Autodesk Fusion 360 part; units mm, degrees
note: some values were not read from the file. Chosen so that the rebuilt part matches the saved one: a direction. Set by a fixed rule: which sketch regions a step uses.
(part 5 of 6)
  spline S19 degree 5 poles (-3.1053, -47.8876) (-3.107, -47.8816) (-3.1103, -47.8695) (-3.1154, -47.8514) (-3.1223, -47.8272) (-3.1309, -47.7972) (-3.1397, -47.7672) (-3.1486, -47.7373) (-3.1576, -47.7075) (-3.1668, -47.6777) (-3.176, -47.6481) (-3.1854, -47.6185) (-3.1949, -47.589) (-3.2046, -47.5596) (-3.2143, -47.5303) (-3.2242, -47.5011) (-3.2342, -47.472) (-3.2443, -47.4429) (-3.2546, -47.414) (-3.2649, -47.3851) (-3.2754, -47.3563) (-3.2861, -47.3277) (-3.2968, -47.2991) (-3.3077, -47.2706) (-3.3187, -47.2422) (-3.3298, -47.2139) (-3.3411, -47.1858) (-3.3525, -47.1577) (-3.364, -47.1297) (-3.3756, -47.1018) (-3.3874, -47.074) (-3.3993, -47.0463) (-3.4114, -47.0188) (-3.4236, -46.9913) (-3.4359, -46.964) (-3.4483, -46.9367) (-3.4609, -46.9096) (-3.4736, -46.8826) (-3.4865, -46.8557) (-3.4995, -46.8289) (-3.5126, -46.8023) (-3.5259, -46.7758) (-3.5394, -46.7494) (-3.5529, -46.7231) (-3.5667, -46.6969) (-3.5805, -46.6709) (-3.5946, -46.645) (-3.6087, -46.6193) (-3.623, -46.5936) (-3.6375, -46.5682) (-3.6522, -46.5428) (-3.667, -46.5177) (-3.6819, -46.4926) (-3.6971, -46.4678) (-3.7124, -46.4431) (-3.7279, -46.4186) (-3.7436, -46.3942) (-3.7594, -46.3699) (-3.7753, -46.3458) (-3.7915, -46.3219) (-3.8078, -46.2982) (-3.8245, -46.2748) (-3.8414, -46.2516) (-3.8585, -46.2287) (-3.8759, -46.2061) (-3.8935, -46.1836) (-3.9112, -46.1612) (-3.9291, -46.139) (-3.9471, -46.117) (-3.9654, -46.0954) (-3.9844, -46.0743) (-4.0001, -46.0581) (-4.0123, -46.0463) (-4.0207, -46.0387) (-4.0249, -46.0349) knots -1 -1 -1 -1 -1 -1 -0.98571429 -0.97142857 -0.95714286 -0.94285714 -0.92857143 -0.91428571 -0.9 -0.88571429 -0.87142857 -0.85714286 -0.84285714 -0.82857143 -0.81428571 -0.8 -0.78571429 -0.77142857 -0.75714286 -0.74285714 -0.72857143 -0.71428571 -0.7 -0.68571429 -0.67142857 -0.65714286 -0.64285714 -0.62857143 -0.61428571 -0.6 -0.58571429 -0.57142857 -0.55714286 -0.54285714 -0.52857143 -0.51428571 -0.5 -0.48571429 -0.47142857 -0.45714286 -0.44285714 -0.42857143 -0.41428571 -0.4 -0.38571429 -0.37142857 -0.35714286 -0.34285714 -0.32857143 -0.31428571 -0.3 -0.28571429 -0.27142857 -0.25714286 -0.24285714 -0.22857143 -0.21428571 -0.2 -0.18571429 -0.17142857 -0.15714286 -0.14285714 -0.12857143 -0.11428571 -0.1 -0.08571429 -0.07142857 -0.05714286 -0.04285714 -0.02857143 -0.01428571 0 0 0 0 0 0
  line L19 (-4.0249, -46.0349) -> (-4.3883, -45.7105)
  arc A39 (-4.397, -45.57) -> (-4.3883, -45.7105) centre (-4.3217, -45.6359) ccw
  arc A40 (-4.397, -45.57) -> (-3.7561, -44.7724) centre (-13.5, -37.5997) ccw
  arc A41 (-3.6171, -44.7506) -> (-3.7561, -44.7724) centre (-3.6756, -44.8317) ccw
  line L20 (-3.6171, -44.7506) -> (-3.222, -45.0357)
  spline S20 degree 5 poles (-3.222, -45.0357) (-3.2174, -45.039) (-3.2081, -45.0455) (-3.194, -45.0549) (-3.1748, -45.0668) (-3.1502, -45.0807) (-3.1251, -45.094) (-3.0997, -45.1068) (-3.0742, -45.1194) (-3.0485, -45.1319) (-3.0228, -45.1442) (-2.9969, -45.1563) (-2.9708, -45.1682) (-2.9446, -45.1797) (-2.9181, -45.1909) (-2.8915, -45.2018) (-2.8646, -45.2124) (-2.8377, -45.2228) (-2.8106, -45.233) (-2.7834, -45.243) (-2.7561, -45.2529) (-2.7287, -45.2625) (-2.7012, -45.272) (-2.6735, -45.2812) (-2.6457, -45.2902) (-2.6178, -45.2991) (-2.5898, -45.3077) (-2.5617, -45.3162) (-2.5335, -45.3245) (-2.5052, -45.3326) (-2.4768, -45.3405) (-2.4483, -45.3483) (-2.4198, -45.3559) (-2.3911, -45.3633) (-2.3623, -45.3706) (-2.3335, -45.3777) (-2.3045, -45.3846) (-2.2755, -45.3914) (-2.2464, -45.398) (-2.2172, -45.4044) (-2.1879, -45.4107) (-2.1585, -45.4169) (-2.1291, -45.4229) (-2.0996, -45.4287) (-2.07, -45.4344) (-2.0403, -45.4399) (-2.0106, -45.4452) (-1.9808, -45.4505) (-1.9509, -45.4555) (-1.921, -45.4605) (-1.8909, -45.4652) (-1.8608, -45.4699) (-1.8307, -45.4744) (-1.8005, -45.4787) (-1.7702, -45.4829) (-1.7398, -45.487) (-1.7094, -45.4909) (-1.6789, -45.4946) (-1.6484, -45.4983) (-1.6178, -45.5018) (-1.5871, -45.5051) (-1.5564, -45.5083) (-1.5256, -45.5114) (-1.4948, -45.5143) (-1.4639, -45.5171) (-1.4329, -45.5198) (-1.4019, -45.5223) (-1.3709, -45.5247) (-1.3397, -45.527) (-1.3086, -45.5291) (-1.2773, -45.5311) (-1.2523, -45.5326) (-1.2335, -45.5336) (-1.221, -45.5343) (-1.2147, -45.5346) knots 0 0 0 0 0 0 0.01428571 0.02857143 0.04285714 0.05714286 0.07142857 0.08571429 0.1 0.11428571 0.12857143 0.14285714 0.15714286 0.17142857 0.18571429 0.2 0.21428571 0.22857143 0.24285714 0.25714286 0.27142857 0.28571429 0.3 0.31428571 0.32857143 0.34285714 0.35714286 0.37142857 0.38571429 0.4 0.41428571 0.42857143 0.44285714 0.45714286 0.47142857 0.48571429 0.5 0.51428571 0.52857143 0.54285714 0.55714286 0.57142857 0.58571429 0.6 0.61428571 0.62857143 0.64285714 0.65714286 0.67142857 0.68571429 0.7 0.71428571 0.72857143 0.74285714 0.75714286 0.77142857 0.78571429 0.8 0.81428571 0.82857143 0.84285714 0.85714286 0.87142857 0.88571429 0.9 0.91428571 0.92857143 0.94285714 0.95714286 0.97142857 0.98571429 1 1 1 1 1 1
  arc A42 (-1.2147, -45.5346) -> (-0.7968, -44.8467) centre (-13.5, -37.5997) ccw
  spline S21 degree 5 poles (-0.7968, -44.8467) (-0.8, -44.8413) (-0.8064, -44.8305) (-0.8159, -44.8143) (-0.8288, -44.7928) (-0.8449, -44.766) (-0.8612, -44.7393) (-0.8775, -44.7127) (-0.894, -44.6863) (-0.9105, -44.6599) (-0.9271, -44.6337) (-0.9438, -44.6075) (-0.9606, -44.5815) (-0.9776, -44.5556) (-0.9946, -44.5298) (-1.0117, -44.5041) (-1.0289, -44.4786) (-1.0462, -44.4532) (-1.0636, -44.4278) (-1.081, -44.4027) (-1.0986, -44.3776) (-1.1163, -44.3526) (-1.1341, -44.3278) (-1.152, -44.3031) (-1.1699, -44.2785) (-1.188, -44.2541) (-1.2062, -44.2298) (-1.2245, -44.2056) (-1.2428, -44.1816) (-1.2613, -44.1576) (-1.2799, -44.1339) (-1.2985, -44.1102) (-1.3173, -44.0867) (-1.3362, -44.0633) (-1.3552, -44.0401) (-1.3742, -44.017) (-1.3934, -43.9941) (-1.4127, -43.9713) (-1.4321, -43.9486) (-1.4516, -43.9261) (-1.4712, -43.9038) (-1.4909, -43.8816) (-1.5107, -43.8596) (-1.5306, -43.8377) (-1.5506, -43.816) (-1.5707, -43.7945) (-1.591, -43.7731) (-1.6113, -43.7519) (-1.6318, -43.7308) (-1.6524, -43.71) (-1.6731, -43.6893) (-1.6939, -43.6688) (-1.7148, -43.6485) (-1.7359, -43.6284) (-1.7571, -43.6086) (-1.7784, -43.5889) (-1.7998, -43.5694) (-1.8214, -43.55) (-1.843, -43.5309) (-1.8648, -43.512) (-1.8867, -43.4933) (-1.9089, -43.475) (-1.9312, -43.457) (-1.9537, -43.4393) (-1.9764, -43.4219) (-1.9992, -43.4048) (-2.0221, -43.3878) (-2.045, -43.3709) (-2.0681, -43.3543) (-2.0915, -43.3382) (-2.1152, -43.3227) (-2.1346, -43.3111) (-2.1495, -43.3029) (-2.1595, -43.2977) (-2.1645, -43.2952) knots -1 -1 -1 -1 -1 -1 -0.98571429 -0.97142857 -0.95714286 -0.94285714 -0.92857143 -0.91428571 -0.9 -0.88571429 -0.87142857 -0.85714286 -0.84285714 -0.82857143 -0.81428571 -0.8 -0.78571429 -0.77142857 -0.75714286 -0.74285714 -0.72857143 -0.71428571 -0.7 -0.68571429 -0.67142857 -0.65714286 -0.64285714 -0.62857143 -0.61428571 -0.6 -0.58571429 -0.57142857 -0.55714286 -0.54285714 -0.52857143 -0.51428571 -0.5 -0.48571429 -0.47142857 -0.45714286 -0.44285714 -0.42857143 -0.41428571 -0.4 -0.38571429 -0.37142857 -0.35714286 -0.34285714 -0.32857143 -0.31428571 -0.3 -0.28571429 -0.27142857 -0.25714286 -0.24285714 -0.22857143 -0.21428571 -0.2 -0.18571429 -0.17142857 -0.15714286 -0.14285714 -0.12857143 -0.11428571 -0.1 -0.08571429 -0.07142857 -0.05714286 -0.04285714 -0.02857143 -0.01428571 0 0 0 0 0 0
  line L21 (-2.1645, -43.2952) -> (-2.5996, -43.0759)
  arc A43 (-2.6443, -42.9424) -> (-2.5996, -43.0759) centre (-2.5546, -42.9866) ccw
  arc A44 (-2.6443, -42.9424) -> (-2.2317, -42.0061) centre (-13.5, -37.5997) ccw
  arc A45 (-2.1031, -41.9491) -> (-2.2317, -42.0061) centre (-2.1386, -42.0425) ccw
  line L22 (-2.1031, -41.9491) -> (-1.6476, -42.1221)
  spline S22 degree 5 poles (-1.6476, -42.1221) (-1.6423, -42.1241) (-1.6317, -42.128) (-1.6157, -42.1335) (-1.594, -42.14) (-1.5666, -42.147) (-1.5389, -42.1534) (-1.5111, -42.1592) (-1.4832, -42.1648) (-1.4552, -42.1702) (-1.4271, -42.1755) (-1.399, -42.1805) (-1.3707, -42.1851) (-1.3424, -42.1895) (-1.3139, -42.1934) (-1.2854, -42.1971) (-1.2567, -42.2004) (-1.228, -42.2034) (-1.1992, -42.2063) (-1.1703, -42.2089) (-1.1414, -42.2114) (-1.1124, -42.2136) (-1.0834, -42.2156) (-1.0543, -42.2174) (-1.0251, -42.2189) (-0.9959, -42.2202) (-0.9666, -42.2213) (-0.9373, -42.2222) (-0.9079, -42.2229) (-0.8785, -42.2234) (-0.849, -42.2238) (-0.8194, -42.2239) (-0.7899, -42.2238) (-0.7602, -42.2236) (-0.7306, -42.2232) (-0.7009, -42.2225) (-0.6711, -42.2218) (-0.6413, -42.2208) (-0.6115, -42.2196) (-0.5816, -42.2183) (-0.5517, -42.2168) (-0.5218, -42.2151) (-0.4918, -42.2133) (-0.4618, -42.2113) (-0.4317, -42.2091) (-0.4016, -42.2067) (-0.3715, -42.2042) (-0.3414, -42.2016) (-0.3112, -42.1987) (-0.281, -42.1957) (-0.2508, -42.1926) (-0.2205, -42.1893) (-0.1902, -42.1858) (-0.1599, -42.1822) (-0.1295, -42.1784) (-0.0992, -42.1744) (-0.0688, -42.1704) (-0.0384, -42.1661) (-0.0079, -42.1617) (0.0225, -42.1572) (0.053, -42.1525) (0.0835, -42.1476) (0.1141, -42.1426) (0.1446, -42.1375) (0.1752, -42.1322) (0.2058, -42.1267) (0.2364, -42.1212) (0.267, -42.1154) (0.2976, -42.1095) (0.3283, -42.1035) (0.359, -42.0974) (0.3835, -42.0923) (0.4019, -42.0885) (0.4142, -42.0859) (0.4204, -42.0846) knots 0 0 0 0 0 0 0.01428571 0.02857143 0.04285714 0.05714286 0.07142857 0.08571429 0.1 0.11428571 0.12857143 0.14285714 0.15714286 0.17142857 0.18571429 0.2 0.21428571 0.22857143 0.24285714 0.25714286 0.27142857 0.28571429 0.3 0.31428571 0.32857143 0.34285714 0.35714286 0.37142857 0.38571429 0.4 0.41428571 0.42857143 0.44285714 0.45714286 0.47142857 0.48571429 0.5 0.51428571 0.52857143 0.54285714 0.55714286 0.57142857 0.58571429 0.6 0.61428571 0.62857143 0.64285714 0.65714286 0.67142857 0.68571429 0.7 0.71428571 0.72857143 0.74285714 0.75714286 0.77142857 0.78571429 0.8 0.81428571 0.82857143 0.84285714 0.85714286 0.87142857 0.88571429 0.9 0.91428571 0.92857143 0.94285714 0.95714286 0.97142857 0.98571429 1 1 1 1 1 1
  arc A46 (0.4204, -42.0846) -> (0.646, -41.312) centre (-13.5, -37.5997) ccw
  spline S23 degree 5 poles (0.646, -41.312) (0.6415, -41.3076) (0.6326, -41.2988) (0.6191, -41.2856) (0.6012, -41.2681) (0.5786, -41.2464) (0.556, -41.2249) (0.5334, -41.2034) (0.5106, -41.1821) (0.4878, -41.1609) (0.465, -41.1399) (0.4421, -41.119) (0.4191, -41.0982) (0.3961, -41.0775) (0.373, -41.057) (0.3498, -41.0367) (0.3266, -41.0164) (0.3033, -40.9963) (0.2799, -40.9764) (0.2565, -40.9566) (0.233, -40.9369) (0.2095, -40.9174) (0.1859, -40.898) (0.1622, -40.8788) (0.1385, -40.8597) (0.1147, -40.8408) (0.0909, -40.822) (0.067, -40.8034) (0.043, -40.7849) (0.019, -40.7666) (-0.0051, -40.7484) (-0.0293, -40.7304) (-0.0535, -40.7126) (-0.0777, -40.6949) (-0.1021, -40.6773) (-0.1265, -40.66) (-0.1509, -40.6428) (-0.1755, -40.6258) (-0.2001, -40.6089) (-0.2247, -40.5922) (-0.2494, -40.5757) (-0.2742, -40.5594) (-0.299, -40.5432) (-0.3239, -40.5273) (-0.3489, -40.5115) (-0.3739, -40.4959) (-0.399, -40.4805) (-0.4241, -40.4652) (-0.4493, -40.4502) (-0.4746, -40.4354) (-0.5, -40.4208) (-0.5254, -40.4064) (-0.5508, -40.3922) (-0.5764, -40.3782) (-0.602, -40.3645) (-0.6277, -40.351) (-0.6534, -40.3377) (-0.6793, -40.3246) (-0.7051, -40.3117) (-0.7311, -40.2991) (-0.7571, -40.2868) (-0.7832, -40.2748) (-0.8094, -40.2632) (-0.8357, -40.2519) (-0.8621, -40.241) (-0.8886, -40.2303) (-0.9151, -40.2198) (-0.9417, -40.2095) (-0.9683, -40.1995) (-0.995, -40.1899) (-1.0219, -40.1811) (-1.0437, -40.1749) (-1.0601, -40.1709) (-1.0712, -40.1684) (-1.0767, -40.1673) knots -1 -1 -1 -1 -1 -1 -0.98571429 -0.97142857 -0.95714286 -0.94285714 -0.92857143 -0.91428571 -0.9 -0.88571429 -0.87142857 -0.85714286 -0.84285714 -0.82857143 -0.81428571 -0.8 -0.78571429 -0.77142857 -0.75714286 -0.74285714 -0.72857143 -0.71428571 -0.7 -0.68571429 -0.67142857 -0.65714286 -0.64285714 -0.62857143 -0.61428571 -0.6 -0.58571429 -0.57142857 -0.55714286 -0.54285714 -0.52857143 -0.51428571 -0.5 -0.48571429 -0.47142857 -0.45714286 -0.44285714 -0.42857143 -0.41428571 -0.4 -0.38571429 -0.37142857 -0.35714286 -0.34285714 -0.32857143 -0.31428571 -0.3 -0.28571429 -0.27142857 -0.25714286 -0.24285714 -0.22857143 -0.21428571 -0.2 -0.18571429 -0.17142857 -0.15714286 -0.14285714 -0.12857143 -0.11428571 -0.1 -0.08571429 -0.07142857 -0.05714286 -0.04285714 -0.02857143 -0.01428571 0 0 0 0 0 0
  line L23 (-1.0767, -40.1673) -> (-1.5537, -40.068)
  arc A47 (-1.6314, -39.9507) -> (-1.5537, -40.068) centre (-1.5333, -39.9701) ccw
  arc A48 (-1.6314, -39.9507) -> (-1.4752, -38.9395) centre (-13.5, -37.5997) ccw
  arc A49 (-1.3657, -38.8511) -> (-1.4752, -38.9395) centre (-1.3758, -38.9506) ccw
  line L24 (-1.3657, -38.8511) -> (-0.881, -38.9004)
  spline S24 degree 5 poles (-0.881, -38.9004) (-0.8754, -38.901) (-0.8641, -38.902) (-0.8472, -38.9031) (-0.8246, -38.9038) (-0.7963, -38.9035) (-0.7679, -38.9025) (-0.7395, -38.9009) (-0.7111, -38.8991) (-0.6827, -38.8971) (-0.6542, -38.8949) (-0.6257, -38.8924) (-0.5972, -38.8896) (-0.5687, -38.8865) (-0.5402, -38.8829) (-0.5117, -38.879) (-0.4832, -38.8748) (-0.4546, -38.8703) (-0.4261, -38.8656) (-0.3975, -38.8607) (-0.3689, -38.8556) (-0.3404, -38.8502) (-0.3118, -38.8447) (-0.2832, -38.8388) (-0.2547, -38.8328) (-0.2261, -38.8265) (-0.1975, -38.82) (-0.1689, -38.8132) (-0.1404, -38.8063) (-0.1118, -38.7992) (-0.0832, -38.7919) (-0.0547, -38.7844) (-0.0261, -38.7767) (0.0024, -38.7688) (0.031, -38.7607) (0.0595, -38.7524) (0.088, -38.7439) (0.1166, -38.7352) (0.1451, -38.7264) (0.1736, -38.7174) (0.2021, -38.7082) (0.2306, -38.6988) (0.2591, -38.6893) (0.2875, -38.6796) (0.316, -38.6697) (0.3444, -38.6597) (0.3729, -38.6494) (0.4013, -38.6391) (0.4297, -38.6285) (0.4581, -38.6178) (0.4865, -38.6069) (0.5149, -38.5959) (0.5432, -38.5847) (0.5716, -38.5734) (0.5999, -38.5618) (0.6282, -38.5502) (0.6565, -38.5384) (0.6848, -38.5264) (0.7131, -38.5143) (0.7413, -38.502) (0.7696, -38.4896) (0.7978, -38.477) (0.826, -38.4642) (0.8541, -38.4514) (0.8823, -38.4383) (0.9104, -38.4252) (0.9386, -38.4119) (0.9666, -38.3984) (0.9947, -38.3848) (1.0228, -38.371) (1.0508, -38.3571) (1.0732, -38.3459) (1.09, -38.3374) (1.1012, -38.3317) (1.1068, -38.3289) knots 0 0 0 0 0 0 0.01428571 0.02857143 0.04285714 0.05714286 0.07142857 0.08571429 0.1 0.11428571 0.12857143 0.14285714 0.15714286 0.17142857 0.18571429 0.2 0.21428571 0.22857143 0.24285714 0.25714286 0.27142857 0.28571429 0.3 0.31428571 0.32857143 0.34285714 0.35714286 0.37142857 0.38571429 0.4 0.41428571 0.42857143 0.44285714 0.45714286 0.47142857 0.48571429 0.5 0.51428571 0.52857143 0.54285714 0.55714286 0.57142857 0.58571429 0.6 0.61428571 0.62857143 0.64285714 0.65714286 0.67142857 0.68571429 0.7 0.71428571 0.72857143 0.74285714 0.75714286 0.77142857 0.78571429 0.8 0.81428571 0.82857143 0.84285714 0.85714286 0.87142857 0.88571429 0.9 0.91428571 0.92857143 0.94285714 0.95714286 0.97142857 0.98571429 1 1 1 1 1 1
  arc A50 (1.1068, -38.3289) -> (1.1248, -37.5242) centre (-13.5, -37.5997) ccw
  spline S25 degree 5 poles (1.1248, -37.5242) (1.1193, -37.5211) (1.1084, -37.5149) (1.092, -37.5057) (1.0701, -37.4935) (1.0427, -37.4784) (1.0153, -37.4634) (0.9879, -37.4485) (0.9604, -37.4338) (0.9329, -37.4193) (0.9054, -37.4048) (0.8779, -37.3906) (0.8503, -37.3764) (0.8227, -37.3625) (0.7951, -37.3486) (0.7674, -37.335) (0.7398, -37.3214) (0.7121, -37.3081) (0.6843, -37.2948) (0.6566, -37.2818) (0.6288, -37.2688) (0.601, -37.2561) (0.5732, -37.2435) (0.5454, -37.231) (0.5176, -37.2187) (0.4897, -37.2066) (0.4618, -37.1946) (0.4339, -37.1828) (0.4059, -37.1712) (0.378, -37.1597) (0.35, -37.1484) (0.322, -37.1372) (0.294, -37.1263) (0.266, -37.1155) (0.2379, -37.1048) (0.2099, -37.0944) (0.1818, -37.0841) (0.1537, -37.074) (0.1256, -37.0641) (0.0975, -37.0543) (0.0693, -37.0448) (0.0412, -37.0354) (0.013, -37.0263) (-0.0152, -37.0173) (-0.0434, -37.0085) (-0.0716, -36.9999) (-0.0998, -36.9915) (-0.128, -36.9833) (-0.1563, -36.9753) (-0.1845, -36.9675) (-0.2128, -36.96) (-0.2411, -36.9526) (-0.2693, -36.9455) (-0.2976, -36.9387) (-0.3259, -36.9321) (-0.3542, -36.9257) (-0.3825, -36.9195) (-0.4109, -36.9135) (-0.4392, -36.9078) (-0.4675, -36.9023) (-0.4958, -36.8971) (-0.5241, -36.8923) (-0.5525, -36.8879) (-0.5808, -36.8838) (-0.6092, -36.8801) (-0.6375, -36.8766) (-0.6658, -36.8733) (-0.6941, -36.8702) (-0.7224, -36.8674) (-0.7507, -36.8651) (-0.779, -36.8636) (-0.8016, -36.8632) (-0.8185, -36.8636) (-0.8298, -36.8641) (-0.8355, -36.8644) knots -1 -1 -1 -1 -1 -1 -0.98571429 -0.97142857 -0.95714286 -0.94285714 -0.92857143 -0.91428571 -0.9 -0.88571429 -0.87142857 -0.85714286 -0.84285714 -0.82857143 -0.81428571 -0.8 -0.78571429 -0.77142857 -0.75714286 -0.74285714 -0.72857143 -0.71428571 -0.7 -0.68571429 -0.67142857 -0.65714286 -0.64285714 -0.62857143 -0.61428571 -0.6 -0.58571429 -0.57142857 -0.55714286 -0.54285714 -0.52857143 -0.51428571 -0.5 -0.48571429 -0.47142857 -0.45714286 -0.44285714 -0.42857143 -0.41428571 -0.4 -0.38571429 -0.37142857 -0.35714286 -0.34285714 -0.32857143 -0.31428571 -0.3 -0.28571429 -0.27142857 -0.25714286 -0.24285714 -0.22857143 -0.21428571 -0.2 -0.18571429 -0.17142857 -0.15714286 -0.14285714 -0.12857143 -0.11428571 -0.1 -0.08571429 -0.07142857 -0.05714286 -0.04285714 -0.02857143 -0.01428571 0 0 0 0 0 0
  line L25 (-0.8355, -36.8644) -> (-1.3219, -36.892)
  arc A51 (-1.4273, -36.7988) -> (-1.3219, -36.892) centre (-1.3276, -36.7921) ccw
  arc A52 (-1.4273, -36.7988) -> (-1.5382, -35.7816) centre (-13.5, -37.5997) ccw
  arc A53 (-1.4553, -35.6679) -> (-1.5382, -35.7816) centre (-1.4393, -35.7666) ccw
  line L26 (-1.4553, -35.6679) -> (-0.9743, -35.5901)
  spline S26 degree 5 poles (-0.9743, -35.5901) (-0.9688, -35.5892) (-0.9576, -35.5872) (-0.941, -35.5839) (-0.919, -35.5787) (-0.8917, -35.5711) (-0.8646, -35.5628) (-0.8376, -35.5539) (-0.8106, -35.5448) (-0.7836, -35.5355) (-0.7567, -35.526) (-0.7298, -35.5162) (-0.703, -35.5062) (-0.6763, -35.4958) (-0.6497, -35.485) (-0.6232, -35.4738) (-0.5967, -35.4624) (-0.5703, -35.4506) (-0.5439, -35.4387) (-0.5176, -35.4266) (-0.4913, -35.4142) (-0.4651, -35.4017) (-0.439, -35.3889) (-0.4129, -35.3759) (-0.3868, -35.3626) (-0.3609, -35.3491) (-0.335, -35.3355) (-0.3091, -35.3216) (-0.2833, -35.3075) (-0.2576, -35.2932) (-0.2319, -35.2787) (-0.2062, -35.2641) (-0.1806, -35.2493) (-0.1551, -35.2342) (-0.1296, -35.219) (-0.1042, -35.2036) (-0.0788, -35.1881) (-0.0535, -35.1723) (-0.0283, -35.1564) (-0.0031, -35.1403) (0.0221, -35.1241) (0.0472, -35.1077) (0.0722, -35.0911) (0.0972, -35.0743) (0.1222, -35.0574) (0.147, -35.0403) (0.1719, -35.0231) (0.1966, -35.0057) (0.2214, -34.9882) (0.246, -34.9705) (0.2706, -34.9526) (0.2952, -34.9346) (0.3197, -34.9165) (0.3441, -34.8982) (0.3685, -34.8797) (0.3928, -34.8611) (0.4171, -34.8424) (0.4413, -34.8235) (0.4655, -34.8045) (0.4896, -34.7853) (0.5136, -34.766) (0.5376, -34.7465) (0.5616, -34.727) (0.5855, -34.7072) (0.6093, -34.6874) (0.6331, -34.6673) (0.6568, -34.6472) (0.6804, -34.6269) (0.704, -34.6065) (0.7276, -34.586) (0.751, -34.5653) (0.7698, -34.5487) (0.7838, -34.5361) (0.7932, -34.5277) (0.7978, -34.5235) knots 0 0 0 0 0 0 0.01428571 0.02857143 0.04285714 0.05714286 0.07142857 0.08571429 0.1 0.11428571 0.12857143 0.14285714 0.15714286 0.17142857 0.18571429 0.2 0.21428571 0.22857143 0.24285714 0.25714286 0.27142857 0.28571429 0.3 0.31428571 0.32857143 0.34285714 0.35714286 0.37142857 0.38571429 0.4 0.41428571 0.42857143 0.44285714 0.45714286 0.47142857 0.48571429 0.5 0.51428571 0.52857143 0.54285714 0.55714286 0.57142857 0.58571429 0.6 0.61428571 0.62857143 0.64285714 0.65714286 0.67142857 0.68571429 0.7 0.71428571 0.72857143 0.74285714 0.75714286 0.77142857 0.78571429 0.8 0.81428571 0.82857143 0.84285714 0.85714286 0.87142857 0.88571429 0.9 0.91428571 0.92857143 0.94285714 0.95714286 0.97142857 0.98571429 1 1 1 1 1 1
  arc A54 (0.7978, -34.5235) -> (0.6069, -33.7416) centre (-13.5, -37.5997) ccw
  spline S27 degree 5 poles (0.6069, -33.7416) (0.6009, -33.74) (0.5887, -33.7369) (0.5705, -33.7322) (0.5462, -33.7261) (0.5158, -33.7186) (0.4854, -33.7112) (0.4551, -33.7039) (0.4248, -33.6968) (0.3944, -33.6899) (0.3641, -33.6831) (0.3338, -33.6764) (0.3035, -33.6699) (0.2733, -33.6636) (0.243, -33.6574) (0.2128, -33.6513) (0.1825, -33.6454) (0.1523, -33.6396) (0.1221, -33.634) (0.0919, -33.6286) (0.0618, -33.6233) (0.0316, -33.6182) (0.0015, -33.6132) (-0.0286, -33.6084) (-0.0587, -33.6037) (-0.0888, -33.5992) (-0.1188, -33.5949) (-0.1488, -33.5907) (-0.1788, -33.5867) (-0.2088, -33.5828) (-0.2387, -33.5791) (-0.2686, -33.5756) (-0.2985, -33.5722) (-0.3284, -33.5691) (-0.3583, -33.5661) (-0.3881, -33.5632) (-0.4178, -33.5606) (-0.4476, -33.5581) (-0.4773, -33.5558) (-0.507, -33.5536) (-0.5367, -33.5517) (-0.5663, -33.5499) (-0.5959, -33.5484) (-0.6254, -33.547) (-0.6549, -33.5458) (-0.6844, -33.5448) (-0.7138, -33.544) (-0.7432, -33.5434) (-0.7725, -33.543) (-0.8019, -33.5428) (-0.8311, -33.5428) (-0.8603, -33.543) (-0.8895, -33.5435) (-0.9186, -33.5442) (-0.9476, -33.5451) (-0.9766, -33.5463) (-1.0056, -33.5476) (-1.0345, -33.5492) (-1.0633, -33.551) (-1.0921, -33.553) (-1.1208, -33.5553) (-1.1494, -33.558) (-1.1779, -33.5611) (-1.2063, -33.5645) (-1.2346, -33.5682) (-1.2629, -33.5722) (-1.2911, -33.5764) (-1.3193, -33.5807) (-1.3473, -33.5853) (-1.3753, -33.5904) (-1.403, -33.5962) (-1.4249, -33.6017) (-1.4412, -33.6065) (-1.452, -33.6099) (-1.4573, -33.6116) knots -1 -1 -1 -1 -1 -1 -0.98571429 -0.97142857 -0.95714286 -0.94285714 -0.92857143 -0.91428571 -0.9 -0.88571429 -0.87142857 -0.85714286 -0.84285714 -0.82857143 -0.81428571 -0.8 -0.78571429 -0.77142857 -0.75714286 -0.74285714 -0.72857143 -0.71428571 -0.7 -0.68571429 -0.67142857 -0.65714286 -0.64285714 -0.62857143 -0.61428571 -0.6 -0.58571429 -0.57142857 -0.55714286 -0.54285714 -0.52857143 -0.51428571 -0.5 -0.48571429 -0.47142857 -0.45714286 -0.44285714 -0.42857143 -0.41428571 -0.4 -0.38571429 -0.37142857 -0.35714286 -0.34285714 -0.32857143 -0.31428571 -0.3 -0.28571429 -0.27142857 -0.25714286 -0.24285714 -0.22857143 -0.21428571 -0.2 -0.18571429 -0.17142857 -0.15714286 -0.14285714 -0.12857143 -0.11428571 -0.1 -0.08571429 -0.07142857 -0.05714286 -0.04285714 -0.02857143 -0.01428571 0 0 0 0 0 0
  line L27 (-1.4573, -33.6116) -> (-1.92, -33.7642)
  arc A55 (-2.046, -33.7014) -> (-1.92, -33.7642) centre (-1.9513, -33.6692) ccw
  arc A56 (-2.046, -33.7014) -> (-2.4163, -32.7476) centre (-13.5, -37.5997) ccw
  arc A57 (-2.3657, -32.6163) -> (-2.4163, -32.7476) centre (-2.3247, -32.7075) ccw
  line L28 (-2.3657, -32.6163) -> (-1.9213, -32.4167)
  spline S28 degree 5 poles (-1.9213, -32.4167) (-1.9161, -32.4143) (-1.9059, -32.4096) (-1.8907, -32.4021) (-1.8708, -32.3913) (-1.8464, -32.377) (-1.8223, -32.3619) (-1.7985, -32.3463) (-1.7748, -32.3305) (-1.7512, -32.3146) (-1.7276, -32.2984) (-1.7042, -32.2821) (-1.6809, -32.2654) (-1.6578, -32.2484) (-1.6349, -32.2311) (-1.6121, -32.2135) (-1.5895, -32.1956) (-1.5671, -32.1774) (-1.5447, -32.1591) (-1.5224, -32.1405) (-1.5002, -32.1218) (-1.4782, -32.1029) (-1.4562, -32.0838) (-1.4344, -32.0644) (-1.4127, -32.0449) (-1.3911, -32.0252) (-1.3696, -32.0052) (-1.3482, -31.9851) (-1.3269, -31.9649) (-1.3058, -31.9444) (-1.2847, -31.9238) (-1.2637, -31.903) (-1.2428, -31.882) (-1.222, -31.8609) (-1.2014, -31.8396) (-1.1808, -31.8182) (-1.1603, -31.7966) (-1.14, -31.7748) (-1.1197, -31.7529) (-1.0995, -31.7309) (-1.0794, -31.7087) (-1.0594, -31.6863) (-1.0395, -31.6638) (-1.0197, -31.6411) (-1, -31.6184) (-0.9804, -31.5954) (-0.9609, -31.5724) (-0.9414, -31.5492) (-0.9221, -31.5258) (-0.9029, -31.5023) (-0.8837, -31.4787) (-0.8647, -31.455) (-0.8457, -31.4311) (-0.8268, -31.4071) (-0.808, -31.383) (-0.7894, -31.3587) (-0.7708, -31.3343) (-0.7523, -31.3098) (-0.7338, -31.2852) (-0.7155, -31.2604) (-0.6973, -31.2356) (-0.6791, -31.2106) (-0.6611, -31.1854) (-0.6431, -31.1602) (-0.6253, -31.1348) (-0.6075, -31.1094) (-0.5898, -31.0838) (-0.5722, -31.0581) (-0.5547, -31.0322) (-0.5372, -31.0063) (-0.5199, -30.9803) (-0.5061, -30.9593) (-0.4958, -30.9436) (-0.489, -30.9331) (-0.4855, -30.9278) knots 0 0 0 0 0 0 0.01428571 0.02857143 0.04285714 0.05714286 0.07142857 0.08571429 0.1 0.11428571 0.12857143 0.14285714 0.15714286 0.17142857 0.18571429 0.2 0.21428571 0.22857143 0.24285714 0.25714286 0.27142857 0.28571429 0.3 0.31428571 0.32857143 0.34285714 0.35714286 0.37142857 0.38571429 0.4 0.41428571 0.42857143 0.44285714 0.45714286 0.47142857 0.48571429 0.5 0.51428571 0.52857143 0.54285714 0.55714286 0.57142857 0.58571429 0.6 0.61428571 0.62857143 0.64285714 0.65714286 0.67142857 0.68571429 0.7 0.71428571 0.72857143 0.74285714 0.75714286 0.77142857 0.78571429 0.8 0.81428571 0.82857143 0.84285714 0.85714286 0.87142857 0.88571429 0.9 0.91428571 0.92857143 0.94285714 0.95714286 0.97142857 0.98571429 1 1 1 1 1 1
  arc A58 (-0.4855, -30.9278) -> (-0.8723, -30.2219) centre (-13.5, -37.5997) ccw
  spline S29 degree 5 poles (-0.8723, -30.2219) (-0.8786, -30.222) (-0.8911, -30.2221) (-0.91, -30.2223) (-0.935, -30.2227) (-0.9663, -30.2232) (-0.9975, -30.224) (-1.0287, -30.2248) (-1.0599, -30.2258) (-1.0909, -30.227) (-1.122, -30.2282) (-1.153, -30.2297) (-1.1839, -30.2312) (-1.2148, -30.2329) (-1.2456, -30.2347) (-1.2764, -30.2367) (-1.3072, -30.2388) (-1.3378, -30.2411) (-1.3684, -30.2435) (-1.399, -30.2461) (-1.4295, -30.2488) (-1.46, -30.2516) (-1.4903, -30.2546) (-1.5207, -30.2577) (-1.5509, -30.261) (-1.5811, -30.2644) (-1.6113, -30.268) (-1.6414, -30.2717) (-1.6714, -30.2756) (-1.7013, -30.2797) (-1.7312, -30.2838) (-1.761, -30.2882) (-1.7908, -30.2927) (-1.8204, -30.2974) (-1.85, -30.3022) (-1.8796, -30.3071) (-1.909, -30.3123) (-1.9384, -30.3176) (-1.9677, -30.323) (-1.9969, -30.3287) (-2.0261, -30.3345) (-2.0551, -30.3404) (-2.0841, -30.3466) (-2.113, -30.3529) (-2.1418, -30.3594) (-2.1705, -30.3661) (-2.1992, -30.3729) (-2.2277, -30.3799) (-2.2562, -30.3871) (-2.2845, -30.3945) (-2.3128, -30.4021) (-2.341, -30.4099) (-2.369, -30.4179) (-2.3969, -30.4261) (-2.4247, -30.4345) (-2.4524, -30.4431) (-2.4801, -30.4519) (-2.5076, -30.4609) (-2.535, -30.4701) (-2.5622, -30.4795) (-2.5894, -30.4892) (-2.6163, -30.4992) (-2.643, -30.5095) (-2.6696, -30.5201) (-2.696, -30.5311) (-2.7223, -30.5422) (-2.7484, -30.5536) (-2.7745, -30.565) (-2.8004, -30.5767) (-2.8261, -30.5889) (-2.8513, -30.6017) (-2.8711, -30.6127) (-2.8856, -30.6215) (-2.8951, -30.6276) (-2.8999, -30.6307) knots -1 -1 -1 -1 -1 -1 -0.98571429 -0.97142857 -0.95714286 -0.94285714 -0.92857143 -0.91428571 -0.9 -0.88571429 -0.87142857 -0.85714286 -0.84285714 -0.82857143 -0.81428571 -0.8 -0.78571429 -0.77142857 -0.75714286 -0.74285714 -0.72857143 -0.71428571 -0.7 -0.68571429 -0.67142857 -0.65714286 -0.64285714 -0.62857143 -0.61428571 -0.6 -0.58571429 -0.57142857 -0.55714286 -0.54285714 -0.52857143 -0.51428571 -0.5 -0.48571429 -0.47142857 -0.45714286 -0.44285714 -0.42857143 -0.41428571 -0.4 -0.38571429 -0.37142857 -0.35714286 -0.34285714 -0.32857143 -0.31428571 -0.3 -0.28571429 -0.27142857 -0.25714286 -0.24285714 -0.22857143 -0.21428571 -0.2 -0.18571429 -0.17142857 -0.15714286 -0.14285714 -0.12857143 -0.11428571 -0.1 -0.08571429 -0.07142857 -0.05714286 -0.04285714 -0.02857143 -0.01428571 0 0 0 0 0 0
  line L29 (-2.8999, -30.6307) -> (-3.3073, -30.8978)
  arc A59 (-3.4452, -30.8697) -> (-3.3073, -30.8978) centre (-3.3621, -30.8141) ccw
  arc A60 (-3.4452, -30.8697) -> (-4.0498, -30.0443) centre (-13.5, -37.5997) ccw
  arc A61 (-4.0349, -29.9043) -> (-4.0498, -30.0443) centre (-3.9717, -29.9819) ccw
  line L30 (-4.0349, -29.9043) -> (-3.6573, -29.5965)
  spline S30 degree 5 poles (-3.6573, -29.5965) (-3.6529, -29.5929) (-3.6442, -29.5856) (-3.6315, -29.5745) (-3.615, -29.5589) (-3.5952, -29.5387) (-3.5759, -29.518) (-3.5569, -29.4968) (-3.5381, -29.4754) (-3.5194, -29.4539) (-3.5009, -29.4322) (-3.4825, -29.4103) (-3.4643, -29.3882) (-3.4464, -29.3658) (-3.4287, -29.3431) (-3.4113, -29.3202) (-3.3941, -29.297) (-3.3771, -29.2737) (-3.3602, -29.2502) (-3.3435, -29.2265) (-3.3269, -29.2027) (-3.3105, -29.1787) (-3.2942, -29.1546) (-3.2781, -29.1302) (-3.2622, -29.1058) (-3.2465, -29.0811) (-3.2309, -29.0563) (-3.2154, -29.0313) (-3.2001, -29.0062) (-3.185, -28.981) (-3.1699, -28.9556) (-3.1551, -28.9301) (-3.1403, -28.9045) (-3.1257, -28.8787) (-3.1113, -28.8528) (-3.0969, -28.8267) (-3.0828, -28.8006) (-3.0687, -28.7743) (-3.0548, -28.7479) (-3.041, -28.7213) (-3.0273, -28.6947) (-3.0138, -28.6679) (-3.0004, -28.641) (-2.9872, -28.614) (-2.974, -28.5869) (-2.961, -28.5597) (-2.9481, -28.5324) (-2.9354, -28.5049) (-2.9227, -28.4774) (-2.9102, -28.4497) (-2.8978, -28.422) (-2.8856, -28.3941) (-2.8734, -28.3661) (-2.8614, -28.3381) (-2.8495, -28.3099) (-2.8378, -28.2816) (-2.8261, -28.2533) (-2.8146, -28.2248) (-2.8032, -28.1962) (-2.7919, -28.1676) (-2.7807, -28.1388) (-2.7696, -28.11) (-2.7587, -28.081) (-2.7479, -28.052) (-2.7372, -28.0229) (-2.7266, -27.9937) (-2.7161, -27.9644) (-2.7058, -27.935) (-2.6956, -27.9055) (-2.6854, -27.876) (-2.6754, -27.8463) (-2.6675, -27.8225) (-2.6617, -27.8047) (-2.6578, -27.7927) (-2.6558, -27.7868) knots 0 0 0 0 0 0 0.01428571 0.02857143 0.04285714 0.05714286 0.07142857 0.08571429 0.1 0.11428571 0.12857143 0.14285714 0.15714286 0.17142857 0.18571429 0.2 0.21428571 0.22857143 0.24285714 0.25714286 0.27142857 0.28571429 0.3 0.31428571 0.32857143 0.34285714 0.35714286 0.37142857 0.38571429 0.4 0.41428571 0.42857143 0.44285714 0.45714286 0.47142857 0.48571429 0.5 0.51428571 0.52857143 0.54285714 0.55714286 0.57142857 0.58571429 0.6 0.61428571 0.62857143 0.64285714 0.65714286 0.67142857 0.68571429 0.7 0.71428571 0.72857143 0.74285714 0.75714286 0.77142857 0.78571429 0.8 0.81428571 0.82857143 0.84285714 0.85714286 0.87142857 0.88571429 0.9 0.91428571 0.92857143 0.94285714 0.95714286 0.97142857 0.98571429 1 1 1 1 1 1
  arc A62 (-2.6558, -27.7868) -> (-3.2121, -27.205) centre (-13.5, -37.5997) ccw
  spline S31 degree 5 poles (-3.2121, -27.205) (-3.2181, -27.2067) (-3.2302, -27.2101) (-3.2484, -27.2151) (-3.2725, -27.222) (-3.3025, -27.2306) (-3.3325, -27.2394) (-3.3624, -27.2483) (-3.3922, -27.2573) (-3.422, -27.2665) (-3.4516, -27.2758) (-3.4812, -27.2851) (-3.5107, -27.2947) (-3.5401, -27.3043) (-3.5694, -27.314) (-3.5986, -27.3239) (-3.6277, -27.3339) (-3.6568, -27.344) (-3.6857, -27.3543) (-3.7146, -27.3647) (-3.7434, -27.3752) (-3.772, -27.3858) (-3.8006, -27.3965) (-3.8291, -27.4074) (-3.8575, -27.4184) (-3.8858, -27.4295) (-3.914, -27.4408) (-3.9421, -27.4522) (-3.97, -27.4637) (-3.9979, -27.4754) (-4.0257, -27.4871) (-4.0534, -27.4991) (-4.0809, -27.5111) (-4.1084, -27.5233) (-4.1357, -27.5356) (-4.163, -27.548) (-4.1901, -27.5606) (-4.2171, -27.5734) (-4.244, -27.5862) (-4.2708, -27.5992) (-4.2974, -27.6124) (-4.324, -27.6256) (-4.3504, -27.6391) (-4.3766, -27.6527) (-4.4028, -27.6664) (-4.4288, -27.6803) (-4.4547, -27.6943) (-4.4804, -27.7084) (-4.5061, -27.7228) (-4.5316, -27.7372) (-4.5569, -27.7519) (-4.5821, -27.7667) (-4.6071, -27.7817) (-4.6319, -27.7968) (-4.6566, -27.8121) (-4.6812, -27.8276) (-4.7055, -27.8433) (-4.7298, -27.8591) (-4.7539, -27.875) (-4.7778, -27.8912) (-4.8015, -27.9076) (-4.8249, -27.9242) (-4.8481, -27.9411) (-4.871, -27.9583) (-4.8936, -27.9757) (-4.9161, -27.9932) (-4.9385, -28.0109) (-4.9607, -28.0288) (-4.9827, -28.0468) (-5.0043, -28.0652) (-5.0254, -28.0841) (-5.0416, -28.0998) (-5.0534, -28.112) (-5.061, -28.1204) (-5.0648, -28.1246) knots -1 -1 -1 -1 -1 -1 -0.98571429 -0.97142857 -0.95714286 -0.94285714 -0.92857143 -0.91428571 -0.9 -0.88571429 -0.87142857 -0.85714286 -0.84285714 -0.82857143 -0.81428571 -0.8 -0.78571429 -0.77142857 -0.75714286 -0.74285714 -0.72857143 -0.71428571 -0.7 -0.68571429 -0.67142857 -0.65714286 -0.64285714 -0.62857143 -0.61428571 -0.6 -0.58571429 -0.57142857 -0.55714286 -0.54285714 -0.52857143 -0.51428571 -0.5 -0.48571429 -0.47142857 -0.45714286 -0.44285714 -0.42857143 -0.41428571 -0.4 -0.38571429 -0.37142857 -0.35714286 -0.34285714 -0.32857143 -0.31428571 -0.3 -0.28571429 -0.27142857 -0.25714286 -0.24285714 -0.22857143 -0.21428571 -0.2 -0.18571429 -0.17142857 -0.15714286 -0.14285714 -0.12857143 -0.11428571 -0.1 -0.08571429 -0.07142857 -0.05714286 -0.04285714 -0.02857143 -0.01428571 0 0 0 0 0 0
  line L31 (-5.0648, -28.1246) -> (-5.3892, -28.4881)
  arc A63 (-5.5297, -28.4967) -> (-5.3892, -28.4881) centre (-5.4638, -28.4215) ccw
  arc A64 (-5.5297, -28.4967) -> (-6.3273, -27.8559) centre (-13.5, -37.5997) ccw
  arc A65 (-6.3491, -27.7168) -> (-6.3273, -27.8559) centre (-6.268, -27.7753) ccw
  line L32 (-6.3491, -27.7168) -> (-6.0641, -27.3217)
  spline S32 degree 5 poles (-6.0641, -27.3217) (-6.0607, -27.3171) (-6.0542, -27.3079) (-6.0448, -27.2938) (-6.033, -27.2745) (-6.019, -27.2499) (-6.0058, -27.2248) (-5.9929, -27.1994) (-5.9803, -27.1739) (-5.9678, -27.1482) (-5.9555, -27.1225) (-5.9434, -27.0966) (-5.9315, -27.0706) (-5.92, -27.0443) (-5.9088, -27.0178) (-5.8979, -26.9912) (-5.8873, -26.9643) (-5.8769, -26.9374) (-5.8667, -26.9103) (-5.8567, -26.8831) (-5.8468, -26.8558) (-5.8372, -26.8284) (-5.8277, -26.8009) (-5.8185, -26.7732) (-5.8095, -26.7454) (-5.8006, -26.7176) (-5.792, -26.6896) (-5.7835, -26.6614) (-5.7752, -26.6332) (-5.7671, -26.6049) (-5.7592, -26.5765) (-5.7514, -26.5481) (-5.7438, -26.5195) (-5.7364, -26.4908) (-5.7291, -26.462) (-5.722, -26.4332) (-5.7151, -26.4042) (-5.7083, -26.3752) (-5.7017, -26.3461) (-5.6953, -26.3169) (-5.689, -26.2876) (-5.6828, -26.2582) (-5.6769, -26.2288) (-5.671, -26.1993) (-5.6654, -26.1697) (-5.6598, -26.14) (-5.6545, -26.1103) (-5.6492, -26.0805) (-5.6442, -26.0506) (-5.6393, -26.0207) (-5.6345, -25.9906) (-5.6298, -25.9606) (-5.6254, -25.9304) (-5.621, -25.9002) (-5.6168, -25.8699) (-5.6128, -25.8395) (-5.6088, -25.8091) (-5.6051, -25.7786) (-5.6014, -25.7481) (-5.598, -25.7175) (-5.5946, -25.6868) (-5.5914, -25.6561) (-5.5883, -25.6253) (-5.5854, -25.5945) (-5.5826, -25.5636) (-5.5799, -25.5326) (-5.5774, -25.5016) (-5.575, -25.4706) (-5.5727, -25.4395) (-5.5706, -25.4083) (-5.5686, -25.3771) (-5.5672, -25.352) (-5.5661, -25.3332) (-5.5654, -25.3207) (-5.5651, -25.3144) knots 0 0 0 0 0 0 0.01428571 0.02857143 0.04285714 0.05714286 0.07142857 0.08571429 0.1 0.11428571 0.12857143 0.14285714 0.15714286 0.17142857 0.18571429 0.2 0.21428571 0.22857143 0.24285714 0.25714286 0.27142857 0.28571429 0.3 0.31428571 0.32857143 0.34285714 0.35714286 0.37142857 0.38571429 0.4 0.41428571 0.42857143 0.44285714 0.45714286 0.47142857 0.48571429 0.5 0.51428571 0.52857143 0.54285714 0.55714286 0.57142857 0.58571429 0.6 0.61428571 0.62857143 0.64285714 0.65714286 0.67142857 0.68571429 0.7 0.71428571 0.72857143 0.74285714 0.75714286 0.77142857 0.78571429 0.8 0.81428571 0.82857143 0.84285714 0.85714286 0.87142857 0.88571429 0.9 0.91428571 0.92857143 0.94285714 0.95714286 0.97142857 0.98571429 1 1 1 1 1 1
  arc A66 (-5.5651, -25.3144) -> (-6.253, -24.8965) centre (-13.5, -37.5997) ccw
  spline S33 degree 5 poles (-6.253, -24.8965) (-6.2584, -24.8997) (-6.2692, -24.9061) (-6.2854, -24.9157) (-6.3069, -24.9285) (-6.3337, -24.9447) (-6.3604, -24.9609) (-6.387, -24.9772) (-6.4135, -24.9937) (-6.4398, -25.0102) (-6.4661, -25.0268) (-6.4922, -25.0435) (-6.5182, -25.0604) (-6.5441, -25.0773) (-6.5699, -25.0943) (-6.5956, -25.1114) (-6.6211, -25.1286) (-6.6466, -25.1459) (-6.6719, -25.1633) (-6.6971, -25.1808) (-6.7221, -25.1983) (-6.7471, -25.216) (-6.7719, -25.2338) (-6.7966, -25.2517) (-6.8212, -25.2697) (-6.8456, -25.2877) (-6.8699, -25.3059) (-6.8941, -25.3242) (-6.9182, -25.3426) (-6.9421, -25.361) (-6.9659, -25.3796) (-6.9895, -25.3983) (-7.013, -25.417) (-7.0364, -25.4359) (-7.0596, -25.4549) (-7.0827, -25.4739) (-7.1056, -25.4931) (-7.1284, -25.5124) (-7.1511, -25.5318) (-7.1736, -25.5513) (-7.1959, -25.5709) (-7.2181, -25.5906) (-7.2401, -25.6104) (-7.262, -25.6303) (-7.2837, -25.6503) (-7.3052, -25.6705) (-7.3266, -25.6907) (-7.3478, -25.7111) (-7.3689, -25.7315) (-7.3897, -25.7521) (-7.4104, -25.7728) (-7.4309, -25.7936) (-7.4512, -25.8145) (-7.4713, -25.8356) (-7.4912, -25.8568) (-7.5109, -25.8781) (-7.5304, -25.8995) (-7.5497, -25.9211) (-7.5688, -25.9427) (-7.5877, -25.9645) (-7.6064, -25.9865) (-7.6247, -26.0086) (-7.6427, -26.0309) (-7.6604, -26.0534) (-7.6778, -26.0761) (-7.695, -26.0989) (-7.712, -26.1218) (-7.7288, -26.1448) (-7.7454, -26.1679) (-7.7615, -26.1912) (-7.777, -26.2149) (-7.7886, -26.2343) (-7.7968, -26.2492) (-7.802, -26.2592) (-7.8045, -26.2643) knots -1 -1 -1 -1 -1 -1 -0.98571429 -0.97142857 -0.95714286 -0.94285714 -0.92857143 -0.91428571 -0.9 -0.88571429 -0.87142857 -0.85714286 -0.84285714 -0.82857143 -0.81428571 -0.8 -0.78571429 -0.77142857 -0.75714286 -0.74285714 -0.72857143 -0.71428571 -0.7 -0.68571429 -0.67142857 -0.65714286 -0.64285714 -0.62857143 -0.61428571 -0.6 -0.58571429 -0.57142857 -0.55714286 -0.54285714 -0.52857143 -0.51428571 -0.5 -0.48571429 -0.47142857 -0.45714286 -0.44285714 -0.42857143 -0.41428571 -0.4 -0.38571429 -0.37142857 -0.35714286 -0.34285714 -0.32857143 -0.31428571 -0.3 -0.28571429 -0.27142857 -0.25714286 -0.24285714 -0.22857143 -0.21428571 -0.2 -0.18571429 -0.17142857 -0.15714286 -0.14285714 -0.12857143 -0.11428571 -0.1 -0.08571429 -0.07142857 -0.05714286 -0.04285714 -0.02857143 -0.01428571 0 0 0 0 0 0
  line L33 (-7.8045, -26.2643) -> (-8.0239, -26.6993)
  arc A67 (-8.1573, -26.744) -> (-8.0239, -26.6993) centre (-8.1132, -26.6543) ccw
  arc A68 (-8.1573, -26.744) -> (-9.0936, -26.3314) centre (-13.5, -37.5997) ccw
  arc A69 (-9.1507, -26.2028) -> (-9.0936, -26.3314) centre (-9.0572, -26.2383) ccw
  line L34 (-9.1507, -26.2028) -> (-8.9776, -25.7474)
  spline S34 degree 5 poles (-8.9776, -25.7474) (-8.9756, -25.7421) (-8.9717, -25.7314) (-8.9662, -25.7154) (-8.9598, -25.6937) (-8.9527, -25.6663) (-8.9463, -25.6386) (-8.9405, -25.6108) (-8.9349, -25.5829) (-8.9295, -25.5549) (-8.9243, -25.5268) (-8.9193, -25.4987) (-8.9146, -25.4705) (-8.9102, -25.4421) (-8.9063, -25.4137) (-8.9027, -25.3851) (-8.8993, -25.3564) (-8.8963, -25.3277) (-8.8934, -25.2989) (-8.8908, -25.27) (-8.8883, -25.2411) (-8.8861, -25.2122) (-8.8841, -25.1831) (-8.8823, -25.154) (-8.8808, -25.1248) (-8.8795, -25.0956) (-8.8784, -25.0663) (-8.8775, -25.037) (-8.8768, -25.0076) (-8.8763, -24.9782) (-8.876, -24.9487) (-8.8758, -24.9192) (-8.8759, -24.8896) (-8.8761, -24.86) (-8.8765, -24.8303) (-8.8772, -24.8006) (-8.878, -24.7708) (-8.8789, -24.741) (-8.8801, -24.7112) (-8.8814, -24.6813) (-8.8829, -24.6514) (-8.8846, -24.6215) (-8.8864, -24.5915) (-8.8884, -24.5615) (-8.8906, -24.5314) (-8.893, -24.5013) (-8.8955, -24.4712) (-8.8981, -24.4411) (-8.901, -24.4109) (-8.904, -24.3807) (-8.9071, -24.3505) (-8.9104, -24.3202) (-8.9139, -24.2899) (-8.9175, -24.2596) (-8.9213, -24.2293) (-8.9253, -24.1989) (-8.9294, -24.1685) (-8.9336, -24.1381) (-8.938, -24.1076) (-8.9426, -24.0772) (-8.9473, -24.0467) (-8.9521, -24.0162) (-8.9571, -23.9857) (-8.9622, -23.9551) (-8.9675, -23.9245) (-8.973, -23.8939) (-8.9786, -23.8633) (-8.9843, -23.8327) (-8.9902, -23.8021) (-8.9962, -23.7714) (-9.0024, -23.7407) (-9.0074, -23.7162) (-9.0112, -23.6978) (-9.0138, -23.6855) (-9.0151, -23.6793) knots 0 0 0 0 0 0 0.01428571 0.02857143 0.04285714 0.05714286 0.07142857 0.08571429 0.1 0.11428571 0.12857143 0.14285714 0.15714286 0.17142857 0.18571429 0.2 0.21428571 0.22857143 0.24285714 0.25714286 0.27142857 0.28571429 0.3 0.31428571 0.32857143 0.34285714 0.35714286 0.37142857 0.38571429 0.4 0.41428571 0.42857143 0.44285714 0.45714286 0.47142857 0.48571429 0.5 0.51428571 0.52857143 0.54285714 0.55714286 0.57142857 0.58571429 0.6 0.61428571 0.62857143 0.64285714 0.65714286 0.67142857 0.68571429 0.7 0.71428571 0.72857143 0.74285714 0.75714286 0.77142857 0.78571429 0.8 0.81428571 0.82857143 0.84285714 0.85714286 0.87142857 0.88571429 0.9 0.91428571 0.92857143 0.94285714 0.95714286 0.97142857 0.98571429 1 1 1 1 1 1
  arc A70 (-9.0151, -23.6793) -> (-9.7878, -23.4537) centre (-13.5, -37.5997) ccw
  spline S35 degree 5 poles (-9.7878, -23.4537) (-9.7922, -23.4582) (-9.801, -23.4671) (-9.8141, -23.4806) (-9.8316, -23.4986) (-9.8533, -23.5211) (-9.8749, -23.5437) (-9.8963, -23.5664) (-9.9176, -23.5891) (-9.9388, -23.6119) (-9.9598, -23.6347) (-9.9808, -23.6576) (-10.0015, -23.6806) (-10.0222, -23.7037) (-10.0427, -23.7268) (-10.063, -23.7499) (-10.0833, -23.7731) (-10.1034, -23.7964) (-10.1233, -23.8198) (-10.1431, -23.8432) (-10.1628, -23.8667) (-10.1823, -23.8902) (-10.2017, -23.9138) (-10.2209, -23.9375) (-10.24, -23.9612) (-10.2589, -23.985) (-10.2777, -24.0088) (-10.2963, -24.0327) (-10.3148, -24.0567) (-10.3331, -24.0807) (-10.3513, -24.1048) (-10.3693, -24.129) (-10.3872, -24.1532) (-10.4048, -24.1775) (-10.4224, -24.2018) (-10.4397, -24.2262) (-10.4569, -24.2507) (-10.474, -24.2752) (-10.4908, -24.2998) (-10.5075, -24.3244) (-10.524, -24.3491) (-10.5403, -24.3739) (-10.5565, -24.3987) (-10.5725, -24.4236) (-10.5882, -24.4486) (-10.6038, -24.4736) (-10.6192, -24.4987) (-10.6345, -24.5238) (-10.6495, -24.5491) (-10.6643, -24.5743) (-10.679, -24.5997) (-10.6934, -24.6251) (-10.7075, -24.6506) (-10.7215, -24.6761) (-10.7352, -24.7017) (-10.7487, -24.7274) (-10.762, -24.7532) (-10.7751, -24.779) (-10.788, -24.8048) (-10.8006, -24.8308) (-10.8129, -24.8568) (-10.8249, -24.8829) (-10.8365, -24.9091) (-10.8478, -24.9355) (-10.8587, -24.9619) (-10.8694, -24.9883) (-10.8799, -25.0148) (-10.8902, -25.0414) (-10.9003, -25.068) (-10.9098, -25.0947) (-10.9186, -25.1216) (-10.9248, -25.1434) (-10.9288, -25.1598) (-10.9313, -25.1709) (-10.9324, -25.1764) knots -1 -1 -1 -1 -1 -1 -0.98571429 -0.97142857 -0.95714286 -0.94285714 -0.92857143 -0.91428571 -0.9 -0.88571429 -0.87142857 -0.85714286 -0.84285714 -0.82857143 -0.81428571 -0.8 -0.78571429 -0.77142857 -0.75714286 -0.74285714 -0.72857143 -0.71428571 -0.7 -0.68571429 -0.67142857 -0.65714286 -0.64285714 -0.62857143 -0.61428571 -0.6 -0.58571429 -0.57142857 -0.55714286 -0.54285714 -0.52857143 -0.51428571 -0.5 -0.48571429 -0.47142857 -0.45714286 -0.44285714 -0.42857143 -0.41428571 -0.4 -0.38571429 -0.37142857 -0.35714286 -0.34285714 -0.32857143 -0.31428571 -0.3 -0.28571429 -0.27142857 -0.25714286 -0.24285714 -0.22857143 -0.21428571 -0.2 -0.18571429 -0.17142857 -0.15714286 -0.14285714 -0.12857143 -0.11428571 -0.1 -0.08571429 -0.07142857 -0.05714286 -0.04285714 -0.02857143 -0.01428571 0 0 0 0 0 0
  line L35 (-10.9324, -25.1764) -> (-11.0317, -25.6534)
  arc A71 (-11.149, -25.7311) -> (-11.0317, -25.6534) centre (-11.1296, -25.633) ccw
  arc A72 (-11.149, -25.7311) -> (-12.1602, -25.5749) centre (-13.5, -37.5997) ccw
  arc A73 (-12.2486, -25.4654) -> (-12.1602, -25.5749) centre (-12.1491, -25.4755) ccw
  line L36 (-12.2486, -25.4654) -> (-12.1993, -24.9807)
  spline S36 degree 5 poles (-12.1993, -24.9807) (-12.1987, -24.9751) (-12.1977, -24.9638) (-12.1966, -24.9469) (-12.196, -24.9243) (-12.1962, -24.896) (-12.1973, -24.8676) (-12.1988, -24.8392) (-12.2006, -24.8108) (-12.2027, -24.7824) (-12.2049, -24.7539) (-12.2073, -24.7254) (-12.2101, -24.697) (-12.2132, -24.6685) (-12.2168, -24.6399) (-12.2207, -24.6114) (-12.2249, -24.5829) (-12.2294, -24.5543) (-12.2341, -24.5258) (-12.239, -24.4972) (-12.2441, -24.4687) (-12.2495, -24.4401) (-12.2551, -24.4115) (-12.2609, -24.383) (-12.2669, -24.3544) (-12.2732, -24.3258) (-12.2797, -24.2972) (-12.2865, -24.2687) (-12.2934, -24.2401) (-12.3005, -24.2115) (-12.3078, -24.183) (-12.3154, -24.1544) (-12.3231, -24.1258) (-12.331, -24.0973) (-12.3391, -24.0688) (-12.3473, -24.0402) (-12.3558, -24.0117) (-12.3645, -23.9832) (-12.3733, -23.9546) (-12.3823, -23.9261) (-12.3915, -23.8976) (-12.4009, -23.8691) (-12.4104, -23.8407) (-12.4201, -23.8122) (-12.43, -23.7837) (-12.4401, -23.7553) (-12.4503, -23.7268) (-12.4607, -23.6984) (-12.4712, -23.67) (-12.4819, -23.6416) (-12.4928, -23.6132) (-12.5038, -23.5848) (-12.515, -23.5565) (-12.5264, -23.5281) (-12.5379, -23.4998) (-12.5495, -23.4715) (-12.5614, -23.4432) (-12.5733, -23.4149) (-12.5855, -23.3866) (-12.5977, -23.3584) (-12.6102, -23.3302) (-12.6227, -23.3019) (-12.6355, -23.2737) (-12.6484, -23.2456) (-12.6614, -23.2174) (-12.6745, -23.1893) (-12.6879, -23.1612) (-12.7013, -23.1331) (-12.7149, -23.105) (-12.7287, -23.0769) (-12.7426, -23.0489) (-12.7538, -23.0265) (-12.7623, -23.0097) (-12.768, -22.9985) (-12.7708, -22.9929) knots 0 0 0 0 0 0 0.01428571 0.02857143 0.04285714 0.05714286 0.07142857 0.08571429 0.1 0.11428571 0.12857143 0.14285714 0.15714286 0.17142857 0.18571429 0.2 0.21428571 0.22857143 0.24285714 0.25714286 0.27142857 0.28571429 0.3 0.31428571 0.32857143 0.34285714 0.35714286 0.37142857 0.38571429 0.4 0.41428571 0.42857143 0.44285714 0.45714286 0.47142857 0.48571429 0.5 0.51428571 0.52857143 0.54285714 0.55714286 0.57142857 0.58571429 0.6 0.61428571 0.62857143 0.64285714 0.65714286 0.67142857 0.68571429 0.7 0.71428571 0.72857143 0.74285714 0.75714286 0.77142857 0.78571429 0.8 0.81428571 0.82857143 0.84285714 0.85714286 0.87142857 0.88571429 0.9 0.91428571 0.92857143 0.94285714 0.95714286 0.97142857 0.98571429 1 1 1 1 1 1
  arc A74 (-12.7708, -22.9929) -> (-13.5755, -22.9749) centre (-13.5, -37.5997) ccw
  spline S37 degree 5 poles (-13.5755, -22.9749) (-13.5786, -22.9804) (-13.5848, -22.9913) (-13.594, -23.0077) (-13.6062, -23.0296) (-13.6214, -23.057) (-13.6363, -23.0844) (-13.6512, -23.1118) (-13.6659, -23.1393) (-13.6805, -23.1668) (-13.6949, -23.1943) (-13.7091, -23.2219) (-13.7233, -23.2494) (-13.7372, -23.277) (-13.7511, -23.3046) (-13.7648, -23.3323) (-13.7783, -23.36) (-13.7917, -23.3877) (-13.8049, -23.4154) (-13.818, -23.4431) (-13.8309, -23.4709) (-13.8436, -23.4987) (-13.8562, -23.5265) (-13.8687, -23.5543) (-13.881, -23.5822) (-13.8931, -23.61) (-13.9051, -23.6379) (-13.9169, -23.6658) (-13.9285, -23.6938) (-13.94, -23.7217) (-13.9513, -23.7497) (-13.9625, -23.7777) (-13.9734, -23.8057) (-13.9842, -23.8337) (-13.9949, -23.8618) (-14.0053, -23.8898) (-14.0156, -23.9179) (-14.0257, -23.946) (-14.0356, -23.9741) (-14.0454, -24.0022) (-14.0549, -24.0304) (-14.0643, -24.0585) (-14.0735, -24.0867) (-14.0824, -24.1149) (-14.0912, -24.1431) (-14.0998, -24.1713) (-14.1082, -24.1995) (-14.1164, -24.2277) (-14.1244, -24.256) (-14.1322, -24.2842) (-14.1397, -24.3125) (-14.1471, -24.3408) (-14.1542, -24.3691) (-14.161, -24.3973) (-14.1676, -24.4256) (-14.174, -24.4539) (-14.1802, -24.4823) (-14.1862, -24.5106) (-14.1919, -24.5389) (-14.1974, -24.5672) (-14.2026, -24.5955) (-14.2074, -24.6239) (-14.2118, -24.6522) (-14.2159, -24.6805) (-14.2196, -24.7089) (-14.2231, -24.7372) (-14.2264, -24.7655) (-14.2295, -24.7938) (-14.2323, -24.8221) (-14.2346, -24.8504) (-14.2361, -24.8787) (-14.2365, -24.9013) (-14.2361, -24.9182) (-14.2356, -24.9295) (-14.2353, -24.9352) knots -1 -1 -1 -1 -1 -1 -0.98571429 -0.97142857 -0.95714286 -0.94285714 -0.92857143 -0.91428571 -0.9 -0.88571429 -0.87142857 -0.85714286 -0.84285714 -0.82857143 -0.81428571 -0.8 -0.78571429 -0.77142857 -0.75714286 -0.74285714 -0.72857143 -0.71428571 -0.7 -0.68571429 -0.67142857 -0.65714286 -0.64285714 -0.62857143 -0.61428571 -0.6 -0.58571429 -0.57142857 -0.55714286 -0.54285714 -0.52857143 -0.51428571 -0.5 -0.48571429 -0.47142857 -0.45714286 -0.44285714 -0.42857143 -0.41428571 -0.4 -0.38571429 -0.37142857 -0.35714286 -0.34285714 -0.32857143 -0.31428571 -0.3 -0.28571429 -0.27142857 -0.25714286 -0.24285714 -0.22857143 -0.21428571 -0.2 -0.18571429 -0.17142857 -0.15714286 -0.14285714 -0.12857143 -0.11428571 -0.1 -0.08571429 -0.07142857 -0.05714286 -0.04285714 -0.02857143 -0.01428571 0 0 0 0 0 0
  line L37 (-14.2353, -24.9352) -> (-14.2077, -25.4216)
  arc A75 (-14.3009, -25.5271) -> (-14.2077, -25.4216) centre (-14.3076, -25.4273) ccw
  arc A76 (-14.3009, -25.5271) -> (-15.3181, -25.6379) centre (-13.5, -37.5997) ccw
  arc A77 (-15.4318, -25.555) -> (-15.3181, -25.6379) centre (-15.3331, -25.539) ccw
  line L38 (-15.4318, -25.555) -> (-15.5097, -25.0741)